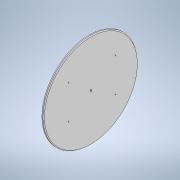
# Autodesk Inventor part: Rotating Base
Saved by Autodesk Inventor 2020.2 (Build 242310000, 310)
## iProperties
Created: 2020-03-31
Part Number: Rotating Base
Material: Generic
Document SubType Name: Modeling
Designer: Amaan Khalid
Density: 1 g/cm^3
Appearance: Default
Author: Amaan Khalid
Autodesk Inventor part; units mm, degrees
ref_plane "YZ Plane" through (0, 0, 0) normal (1, 0, 0) x (0, 1, 0)
ref_plane "XZ Plane" through (0, 0, 0) normal (0, 1, 0) x (-1, 0, 0)
ref_plane "XY Plane" through (0, 0, 0) normal (0, 0, 1) x (1, 0, 0)
sketch "Sketch1" plane through (0, 0, 0) normal (1, 0, 0) x (0, 1, 0)
  circle A0 centre (-42.0801, -52.5105) radius 133.35
  dimension "d38" = 266.7
  constraints: 1 centre point
  measures "d38" diameter of A0
extrude "Extrusion1" add sketch "Sketch1" along normal blind 5.08
fillet "Fillet1" radius 2.286 1 edges at (5.08, -175.4301, -52.5105)
sketch "Sketch2" plane through (5.08, -42.0801, -52.5105) normal (1, 0, 0) x (0, 0, -1)
  line L0 (0.865, -2.45) -> (-0.865, -2.45)
  line L1 (-1.5, -1.815) -> (-1.5, 1.815)
  line L2 (-0.865, 2.45) -> (0.865, 2.45)
  line L3 (1.5, 1.815) -> (1.5, -1.815)
  line L4 (1.5, -2.45) -> (-1.5, 2.45) construction
  line L5 (-1.5, -2.45) -> (1.5, 2.45) construction
  arc A0 (-0.865, 2.45) -> (-1.5, 1.815) centre (-0.865, 1.815) ccw
  arc A1 (1.5, 1.815) -> (0.865, 2.45) centre (0.865, 1.815) ccw
  arc A2 (-1.5, -1.815) -> (-0.865, -2.45) centre (-0.865, -1.815) ccw
  arc A3 (0.865, -2.45) -> (1.5, -1.815) centre (0.865, -1.815) ccw
  point P0 (-52.5105, 42.0801)
  point P1 (0, 0)
  constraints: 12 end point, 8 point on circle, 8 point on line, 8 tangent, 4 centre point, 3 equal radius, 2 midpoint, 2 parallel, 1 horizontal, 1 perpendicular
extrude "Extrusion3" cut sketch "Sketch2" against normal blind 5.08
sketch "Sketch4" plane through (5.08, -42.0801, -52.5105) normal (1, 0, 0) x (0, 0, -1)
  circle A0 centre (-63.4701, -44.45) radius 1.27
  circle A1 centre (-63.5, 50.8) radius 1.27
  circle A2 centre (69.85, 50.8239) radius 1.27
  circle A3 centre (69.8799, -44.4261) radius 1.27
  point P0 (-52.5105, 42.0801)
  constraints: 4 centre point
extrude "Extrusion5" cut sketch "Sketch4" against normal through all
body "Solid1"
